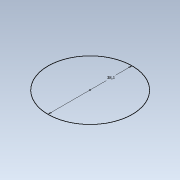
# Autodesk Inventor part: Eje cardan
Saved by Autodesk Inventor 2021 (Build 250183000, 183)
## iProperties
Created: 2021-08-20
Part Number: Eje cardan
Material: Generic
Document SubType Name: Modeling
Designer: Andrés Holguín
Density: 1 g/cm^3
Appearance: Default
Author: Andrés Holguín
Autodesk Inventor part; units mm, degrees
ref_plane "YZ Plane" through (0, 0, 0) normal (1, 0, 0) x (0, 1, 0)
ref_plane "XZ Plane" through (0, 0, 0) normal (0, 1, 0) x (-1, 0, 0)
ref_plane "XY Plane" through (0, 0, 0) normal (0, 0, 1) x (1, 0, 0)
sketch "Sketch1" plane through (0, 0, 0) normal (0, 1, 0) x (-1, 0, 0)
  circle A0 centre (0, 0) radius 19.05
  dimension "d0" = 38.1
  constraints: 1 centre point, 1 coincident
  measures "d0" diameter of A0
extrude "Extrusion1" add sketch "Sketch1" along normal blind 63.5
thread "Thread1" size "1 1/2-6 UNC" class "2A" standard "ANSI Unified Screw Threads" length 50.8
body "Solid1"
